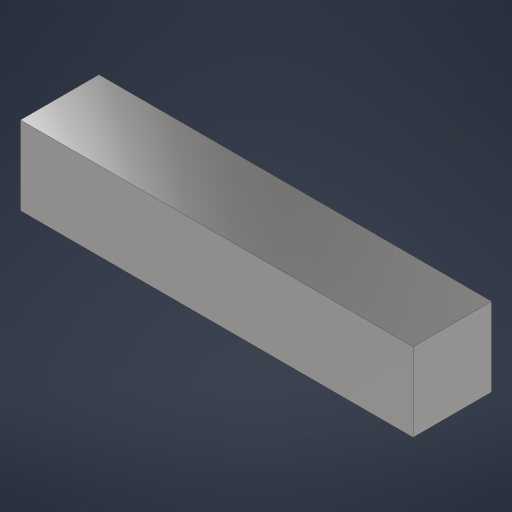
# Autodesk Inventor part: weight60
Saved by Autodesk Inventor 2023 (Build 270158000, 158)
## iProperties
Created: 2022-07-09
Part Number: weight60
Material: Stainless Steel
Document SubType Name: Modeling
Designer: x43dn
Density: 8 g/cm^3
Appearance: Semi-Polished
Author: x43dn
Autodesk Inventor part; units mm, degrees
ref_plane "YZ Plane" through (0, 0, 0) normal (1, 0, 0) x (0, 1, 0)
ref_plane "XZ Plane" through (0, 0, 0) normal (0, 1, 0) x (-1, 0, 0)
ref_plane "XY Plane" through (0, 0, 0) normal (0, 0, 1) x (1, 0, 0)
sketch "Sketch1" plane through (0, 0, 0) normal (1, 0, 0) x (0, 1, 0)
  line L0 (0, 0) -> (12, 0)
  line L1 (12, 0) -> (12, -12)
  line L2 (12, -12) -> (0, -12)
  line L3 (0, -12) -> (0, 0)
  dimension "d0" = 12
  dimension "d1" = 12
  constraints: 8 end point, 2 parallel, 1 horizontal, 1 perpendicular
  measures "d0" distance of L1.end L2.end
  measures "d1" distance of L0.end L1.end
extrude "Extrusion1" add sketch "Sketch1" along normal blind 60
body "Solid1"
